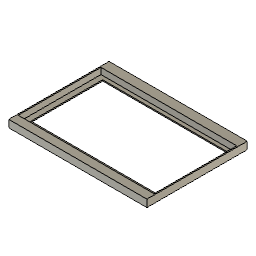
UIv3 (Autodesk Fusion 360 archive; units mm, degrees)
design "displayCasev4"
Autodesk Fusion 360 part; units mm, degrees
sketch "Sketch1" plane through (0, 0, 0) normal (0, 0, 1) x (1, 0, 0)
  line L0 (0, 0) -> (169.51, 0)
  line L1 (169.51, 0) -> (169.51, 124.6)
  line L2 (169.51, 124.6) -> (0, 124.6)
  line L3 (0, 124.6) -> (0, 0)
  dimension "d1" = 169.51
  dimension "d2" = 124.6
  constraint horizontal L0
  constraint vertical L1
  constraint horizontal L2
  constraint vertical L3
  constraint coincident L0.start L3.end
  measures "d1" distance of L0.start L0.end
  measures "d2" distance of L0.start L2.end
extrude "Extrude1" add sketch "Sketch1" along normal blind 9.2 makes body 1
sketch "Sketch2" plane through (0, 0, 9.2) normal (0, 0, 1) x (-1, 0, 0)
  line L0 (0, -124.6) -> (0, 0)
  line L1 (0, 0) -> (-169.51, 0)
  line L2 (-169.51, 0) -> (-169.51, -124.6)
  line L3 (-169.51, -124.6) -> (0, -124.6)
  line L4 (-1.5, -10.3) -> (-168.01, -10.3)
  line L5 (-168.01, -10.3) -> (-168.01, -113)
  line L6 (-168.01, -113) -> (-1.5, -113)
  line L7 (-1.5, -113) -> (-1.5, -10.3)
  dimension "d5" = 1.5
  dimension "d6" = 1.5
  dimension "d7" = 11.6
  dimension "d8" = 10.3
  constraint horizontal L4
  constraint vertical L5
  constraint horizontal L6
  constraint vertical L7
  measures "d5" distance of L0 L7
  measures "d6" distance of L2 L5
  measures "d7" distance of L3 L6
  measures "d8" distance of L1 L4
extrude "Extrude2" cut sketch "Sketch2" against normal blind 7.6 contours L4 L5 L6 L7 bodies 1
sketch "Sketch3" plane through (0, 0, 1.6) normal (0, 0, 1) x (-1, 0, 0)
  line L0 (-1.5, -113) -> (-1.5, -10.3)
  line L1 (-1.5, -10.3) -> (-168.01, -10.3)
  line L2 (-168.01, -10.3) -> (-168.01, -113)
  line L3 (-168.01, -113) -> (-1.5, -113)
  line L4 (-8.2, -19.7) -> (-163.91, -19.7)
  line L5 (-163.91, -19.7) -> (-163.91, -105.62)
  line L6 (-163.91, -105.62) -> (-8.2, -105.62)
  line L7 (-8.2, -105.62) -> (-8.2, -19.7)
  dimension "d12" = 85.92
  dimension "d13" = 9.4
  dimension "d14" = 6.7
  dimension "d15" = 4.1
  constraint horizontal L4
  constraint vertical L5
  constraint horizontal L6
  constraint vertical L7
  measures "d12" distance of L4.start L6.end
  measures "d13" distance of L1 L4
  measures "d14" distance of L0 L7
  measures "d15" distance of L2 L5
extrude "Extrude3" cut sketch "Sketch3" against normal blind 1.6 contours L4 L5 L6 L7 bodies 1
extrude "Extrude4" cut 1 faces at (59.2367, 13.4333, 1.6) along direction (0, 0, -1) blind 0.1 on bodies 1 bodies 1
sketch "Sketch4" plane through (0, 0, 1.5) normal (0, 0, 1) x (-1, 0, 0)
  line L0 (-163.91, -19.7) -> (-8.2, -19.7)
  line L1 (-8.2, -19.7) -> (-8.2, -105.62)
  line L2 (-8.2, -105.62) -> (-163.91, -105.62)
  line L3 (-163.91, -105.62) -> (-163.91, -19.7)
  line L4 (-1.5, -113) -> (-1.5, -10.3)
  line L5 (-1.5, -10.3) -> (-168.01, -10.3)
  line L6 (-168.01, -10.3) -> (-168.01, -113)
  line L7 (-168.01, -113) -> (-1.5, -113)
  line L8 (-8.2, -105.62) -> (-163.9, -105.62)
  line L9 (-163.9, -105.62) -> (-163.9, -108.4)
  line L10 (-163.9, -108.4) -> (-8.2, -108.4)
  line L11 (-8.2, -108.4) -> (-8.2, -105.62)
  dimension "d20" = 4.6
  dimension "d21" = 155.7
  constraint horizontal L8
  constraint vertical L9
  constraint horizontal L10
  constraint vertical L11
  constraint coincident L1.end L2.start
  measures "d20" distance of L7 L10
  measures "d21" distance of L9.end L10.end
extrude "Extrude5" cut sketch "Sketch4" against normal blind 1.5 contours L2 L8 L9 L10 L11 bodies 1
ref_plane "WorkPlane1" through (90, 0, 0) normal (1, 0, 0) x (0, 1, 0)
split "Split1" by plane through (90, 0, 0) normal (1, 0, 0) bodies 1 makes body 2 at (141.14, 6.5667, 0)
move_body "Move1" bodies 2 to x (1, 0, 0) y (0, 1, 0) z (0, 0, 1) at (2, 0, 0)
extrude "Extrude6" add 2 faces at (90, 3.4333, 3.5667) (90, 120.7333, 3.5667) along direction (1, 0, 0) blind 2 on bodies 1 bodies 1 2
